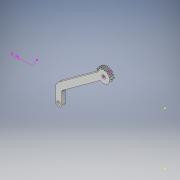
# Autodesk Inventor part: sem2_indexmid-finger2
Saved by Autodesk Inventor 2018 (Build 220112000, 112)
## iProperties
Created: 2017-10-02
Part Number: sem2_indexmid-finger2
Material: Generic
Document SubType Name: Modeling
Designer: rheal
Density: 1 g/cm^3
Appearance: Default
Author: rheal
Autodesk Inventor part; units mm, degrees
note: some values were not read from the file. Chosen so that the rebuilt part matches the saved one: pattern direction of "Circular Pattern2".
ref_plane "YZ Plane" through (0, 0, 0) normal (1, 0, 0) x (0, 1, 0)
ref_plane "XZ Plane" through (0, 0, 0) normal (0, 1, 0) x (-1, 0, 0)
ref_plane "XY Plane" through (0, 0, 0) normal (0, 0, 1) x (1, 0, 0)
sketch "Sketch1" plane through (0, 0, 0) normal (0, 0, 1) x (1, 0, 0)
  arc A0 (-91.6172, 6.0862) -> (-86.0767, 5.7659) centre (-88.8377, 6.0862) ccw
  line L0 (-49.9996, 32.0895) -> (-49.9996, 50.0023) construction
  arc A1 (-46.9559, 41.0355) -> (-49.9996, 50.0023) centre (-49.9996, 45.0023) ccw
  arc A2 (-52.8608, 40.902) -> (-54.8119, 46.3593) centre (-49.9996, 45.0023) ccw
  line L1 (-91.6172, 6.0862) -> (-91.6172, 16.5407)
  arc A3 (-91.6172, 6.0862) -> (-86.0582, 6.0862) centre (-88.8377, 6.0862) ccw
  line L2 (-86.0582, 6.0862) -> (-86.0582, 15.904)
  line L3 (-52.8608, 40.902) -> (-85.2293, 17.4013)
  line L4 (-88.5001, 21.9005) -> (-54.8119, 46.3593)
  arc A4 (-88.5001, 21.9005) -> (-91.6172, 16.5407) centre (-84.2108, 15.8196) ccw
  arc A5 (-85.2293, 17.4013) -> (-86.0582, 15.904) centre (-84.2914, 15.904) ccw
  point P0 (19.05, 139.7)
  point P1 (-45.0073, 44.7246)
  point P2 (-86.0582, 16.8024)
  dimension "d69" = 2.7795
  constraints: 14 point on circle, 10 end point, 6 centre point, 2 tangent, 2 vertical, 1 coincident, 1 point on line
  measures "d69" radius of A0
extrude "Extrusion1" add sketch "Sketch1" along normal blind 3
sketch "Sketch12" plane through (0, 0, 3) normal (0, 0, 1) x (1, 0, 0)
  arc A0 (-91.6172, 6.0862) -> (-86.0582, 6.0862) centre (-88.8377, 6.0862) ccw projected
  circle A1 centre (-88.8377, 6.0862) radius 1.5
  point P0 (-97.2205, 0)
  dimension "d105" = 3
  constraints: 1 centre point, 1 coincident
  measures "d105" diameter of A1
extrude "Extrusion11" cut sketch "Sketch12" against normal through all
sketch "Sketch15" plane through (0, 0, 0) normal (0, 0, -1) x (-1, 0, 0)
  point P0 (0, 0)
sketch "Sketch16" plane through (0, 0, 0) normal (0, 0, -1) x (-1, 0, 0)
  circle A0 centre (50, 45) radius 2.5 projected
  line L0 (50, 45) -> (50, 42.5) construction
  line L1 (50, 45) -> (52.5, 45) construction
  point P0 (0, 0)
  constraints: 4 end point, 2 point on circle, 1 perpendicular, 1 vertical
ref_plane "Work Plane2" through (-50, 45, 0) normal (0, -1, 0) x (1, 0, 0)
sketch "Sketch18" plane through (-50, 45, 0) normal (0, -1, 0) x (1, 0, 0)
  line L0 (0, 0.0908) -> (0, 2.9092) construction
  line L1 (0, 1.5) -> (0, -3.9375) construction
  point P0 (50, 0)
  constraints: 2 end point, 1 midpoint, 1 vertical
sketch "Sketch19" plane through (0, 0, 0) normal (0, 0, -1) x (-1, 0, 0)
  line L0 (40.2723, 49.5) -> (49.7354, 49.2661) construction
  line L1 (49.9819, 50.3977) -> (49.9819, 51.6759) construction
  line L2 (49.9819, 49.9276) -> (49.4819, 49.9276)
  line L3 (49.7319, 51.6759) -> (49.7319, 50.8959)
  arc A0 (49.7319, 50.8959) -> (49.4819, 49.9276) centre (51.3636, 49.9582) ccw
  line L4 (49.7319, 51.6759) -> (49.9819, 51.6759)
  line L5 (59.7277, 49.5) -> (49.7354, 49.2661) construction
  line L6 (49.9819, 49.9276) -> (50.4819, 49.9276)
  line L7 (50.2319, 51.6759) -> (50.2319, 50.8959)
  arc A1 (50.4819, 49.9276) -> (50.2319, 50.8959) centre (48.6002, 49.9582) ccw
  line L8 (50.2319, 51.6759) -> (49.9819, 51.6759)
  point P0 (0, 0)
  point P1 (50, 50)
  dimension "d82" = 1.676
  dimension "d83" = 0.5
  dimension "d84" = 0.25
  dimension "d85" = 1
  dimension "d86" = 0.0746
  constraints: 18 end point, 4 point on circle, 4 symmetric about line, 2 centre point, 1 perpendicular, 1 vertical, 1 other
  measures "d82" distance of point (50, 50) L1.end
  measures "d83" distance of L2.start L2.end
  measures "d84" distance between parallel lines of L1 L3
  measures "d85" distance of L3.end L2.end
  measures "d86" distance of point (50, 50) L2.start
extrude "Extrusion13" add sketch "Sketch19" against normal blind 3
sketch "Sketch20" plane through (0, 0, 0) normal (0, 0, -1) x (-1, 0, 0)
  line L0 (45.7576, 49.2502) -> (46.1486, 48.8898) projected
  line L1 (46.9253, 49.5288) -> (46.647, 49.982) projected
  point P0 (0, 0)
sketch "Sketch21" plane through (0, 0, 0) normal (0, 0, -1) x (-1, 0, 0)
  arc A0 (49.5542, 49.9801) -> (46.9563, 41.0331) centre (50, 45) ccw projected
  circle A1 centre (50, 45) radius 1.5
  point P0 (0, 0)
  dimension "d94" = 3
  constraints: 1 centre point, 1 coincident
  measures "d94" diameter of A1
extrude "Extrusion15" cut sketch "Sketch21" against normal blind 3
pattern_circular "Circular Pattern2" count 10 over 142 about axis through (-50, 45, 0) along (0, 0, -1) of "Extrusion13" both ways yes
body "Solid1"
